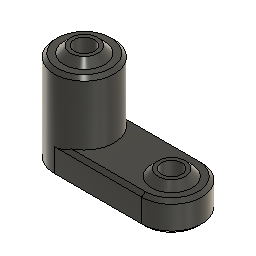
GT2_pulley_upper_support_i2 v3 (Autodesk Fusion 360 design; units mm, degrees)
Autodesk Fusion 360 part; units mm, degrees
sketch "Sketch1" plane through (0, 0, 0) normal (0, 0, 1) x (1, 0, 0)
  circle A0 centre (0, 0) radius 1.525
  circle A1 centre (0, 0) radius 4.5
  circle A2 centre (13.2, 0) radius 1.525
  circle A3 centre (0, 0) radius 2.75
  circle A4 centre (13.2, 0) radius 2.75
  line L0 (0, 4.5) -> (13.2, 4.5)
  line L1 (13.2, -4.5) -> (0, -4.5)
  arc A5 (13.2, -4.5) -> (13.2, 4.5) centre (13.2, 0) ccw
  dimension "d1" = 3.05
  dimension "d2" = 9
  dimension "d3" = 9
  dimension "d4" = 3.05
  dimension "d5" = 5.5
  dimension "d6" = 5.5
  dimension "d7" = 13.2
  constraint coincident A0.centre A1.centre
  constraint concentric A0 A1
  constraint concentric A2 A5
  constraint concentric A1 A3
  constraint concentric A2 A4
  constraint coincident A1 L0.start
  constraint tangent L0 A5
  constraint horizontal L0
  constraint coincident A1 L1.end
  constraint tangent A1 L1
  constraint parallel L0 L1
  measures "d1" diameter of A0
  measures "d2" diameter of A1
  measures "d3" diameter of A5
  measures "d4" diameter of A2
  measures "d5" diameter of A3
  measures "d6" diameter of A4
  measures "d7" distance of A0.centre A2.centre
extrude "Extrude1" add sketch "Sketch1" along normal blind 14 contours A1 | A3
extrude "Extrude2" add sketch "Sketch1" along normal blind 4.5 contours A1 L0 L1 A5 | A4
sketch "Sketch2" plane through (0, 0, 14) normal (0, 0, 1) x (-1, 0, 0)
  circle A0 centre (0, 0) radius 1.525
  circle A1 centre (0, 0) radius 4.5
  circle A2 centre (0, 0) radius 2.05
  dimension "d12" = 4.1
  constraint coincident A0.centre A1.centre
  measures "d12" diameter of A2
extrude "Extrude3" add sketch "Sketch2" along normal blind 1 contours A2
chamfer "Chamfer1" distance 1 angle 45 1 edges at (1.9113, -0.7413, 14)
sketch "Sketch3" plane through (0, 0, 4.5) normal (0, 0, 1) x (-1, 0, 0)
  circle A0 centre (-13.2, 0) radius 1.525
  line L0 (0, 4.5) -> (-13.2, 4.5)
  arc A1 (-13.2, 4.5) -> (-13.2, -4.5) centre (-13.2, 0) ccw
  line L1 (-13.2, -4.5) -> (0, -4.5)
  arc A2 (0, 4.5) -> (0, -4.5) centre (0, 0) ccw
  circle A3 centre (-13.2, 0) radius 2.05
  dimension "d16" = 4.1
  constraint concentric A0 A3
  measures "d16" diameter of A3
extrude "Extrude4" add sketch "Sketch3" along normal blind 1 contours A3
chamfer "Chamfer2" distance 1 angle 45 1 edges at (15.1113, -0.7413, 4.5)
extrude "Extrude5" cut sketch "Sketch1" along normal blind 1 contours A3 | A4
chamfer "Chamfer3" distance 0.5 angle 45 10 edges at (6.6, -4.5, 0) (17.7, 0, 0) (6.6, 4.5, 0) (-4.5, 0, 0) (10.6361, -0.9944, 0) (-2.5639, -0.9944, 0) (-4.1955, -1.6273, 14) (6.6, -4.5, 4.5) (17.7, 0, 4.5) (6.6, 4.5, 4.5)
